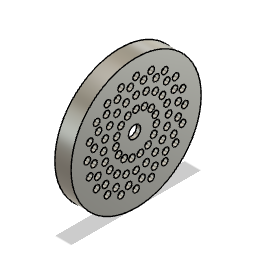
SHAPER_CAE (Autodesk Fusion 360 design; units mm, degrees)
Autodesk Fusion 360 part; units mm, degrees
sketch "Sketch1" plane through (0, 0, 0) normal (1, 0, 0) x (0, 0, -1)
  circle A0 centre (0, 0) radius 80
  circle A1 centre (0, 0) radius 70
  dimension "d1" = 160
  dimension "d2" = 140
  constraint coincident A0.centre A1.centre
  measures "d1" diameter of A0
  measures "d2" diameter of A1
extrude "Extrude1" add sketch "Sketch1" along normal blind 15
thread "Thread1" "ISO Metric profile 140.0 M140x8 6H" major diameter 140.8024 minor diameter 131.8397 pitch 8 angle 60 resizes the face on face at (10, -6.9697, -69.6522)
sketch "Sketch2" plane through (15, 0, 0) normal (1, 0, 0) x (0, 0, -1)
  circle A0 centre (0, 0) radius 65.9198
  circle A1 centre (0, 0) radius 80
  circle A2 centre (0, 0) radius 80
  constraint concentric A0 A2
extrude "Extrude2" add sketch "Sketch2" along normal blind 5 contours A0 | A1 A2
hole "Hole1" at (20, 1.6801, 1.9117) direction (-1, 0, 0) diameter 15 depth 40 tip angle 180
sketch "Sketch3" plane through (20, 0, 0) normal (1, 0, 0) x (0, 0, -1)
  circle A0 centre (-1.9117, 1.6801) radius 7.5
  circle A1 centre (0, 0) radius 80
  point P0 (0, 60)
hole "Hole2" at (20, 60, 0) direction (-1, 0, 0) diameter 8 depth 40 tip angle 180
pattern_circular "C-Pattern1" count 20 over 360 about axis through (1.75, 0, 0) along (1, 0, 0) of "Hole2"
sketch "Sketch4" plane through (20, 0, 0) normal (1, 0, 0) x (0, 0, -1)
  circle A0 centre (18.541, 57.0634) radius 4
  circle A1 centre (35.2671, 48.541) radius 4
  circle A2 centre (48.541, 35.2671) radius 4
  circle A3 centre (57.0634, 18.541) radius 4
  circle A4 centre (60, 0) radius 4
  circle A5 centre (57.0634, -18.541) radius 4
  circle A6 centre (48.541, -35.2671) radius 4
  circle A7 centre (35.2671, -48.541) radius 4
  circle A8 centre (18.541, -57.0634) radius 4
  circle A9 centre (0, -60) radius 4
  circle A10 centre (-18.541, -57.0634) radius 4
  circle A11 centre (-35.2671, -48.541) radius 4
  circle A12 centre (-48.541, -35.2671) radius 4
  circle A13 centre (-57.0634, -18.541) radius 4
  circle A14 centre (-60, 0) radius 4
  circle A15 centre (-57.0634, 18.541) radius 4
  circle A16 centre (-48.541, 35.2671) radius 4
  circle A17 centre (-35.2671, 48.541) radius 4
  circle A18 centre (-18.541, 57.0634) radius 4
  circle A19 centre (0, 60) radius 4
  circle A20 centre (-1.9117, 1.6801) radius 7.5
  circle A21 centre (0, 0) radius 80
  point P0 (-7.2239, 51.8768)
hole "Hole3" at (20, 51.8768, 7.2239) direction (-1, 0, 0) diameter 8 depth 40 tip angle 180
pattern_circular "C-Pattern2" count 20 over 360 about axis through (1.75, 0, 0) along (1, 0, 0) of "Hole3"
sketch "Sketch5" plane through (20, 0, 0) normal (1, 0, 0) x (0, 0, -1)
  circle A0 centre (9.1605, 51.5701) radius 4
  circle A1 centre (24.6482, 46.2153) radius 4
  circle A2 centre (37.7231, 36.3367) radius 4
  circle A3 centre (47.1055, 22.9012) radius 4
  circle A4 centre (51.8768, 7.2239) radius 4
  circle A5 centre (51.5701, -9.1605) radius 4
  circle A6 centre (46.2153, -24.6482) radius 4
  circle A7 centre (36.3367, -37.7231) radius 4
  circle A8 centre (22.9012, -47.1055) radius 4
  circle A9 centre (7.2239, -51.8768) radius 4
  circle A10 centre (-9.1605, -51.5701) radius 4
  circle A11 centre (-24.6482, -46.2153) radius 4
  circle A12 centre (-37.7231, -36.3367) radius 4
  circle A13 centre (-47.1055, -22.9012) radius 4
  circle A14 centre (-51.8768, -7.2239) radius 4
  circle A15 centre (-51.5701, 9.1605) radius 4
  circle A16 centre (-46.2153, 24.6482) radius 4
  circle A17 centre (-36.3367, 37.7231) radius 4
  circle A18 centre (-22.9012, 47.1055) radius 4
  circle A19 centre (-7.2239, 51.8768) radius 4
  circle A20 centre (18.541, 57.0634) radius 4
  circle A21 centre (35.2671, 48.541) radius 4
  circle A22 centre (48.541, 35.2671) radius 4
  circle A23 centre (57.0634, 18.541) radius 4
  circle A24 centre (60, 0) radius 4
  circle A25 centre (57.0634, -18.541) radius 4
  circle A26 centre (48.541, -35.2671) radius 4
  circle A27 centre (35.2671, -48.541) radius 4
  circle A28 centre (18.541, -57.0634) radius 4
  circle A29 centre (0, -60) radius 4
  circle A30 centre (-18.541, -57.0634) radius 4
  circle A31 centre (-35.2671, -48.541) radius 4
  circle A32 centre (-48.541, -35.2671) radius 4
  circle A33 centre (-57.0634, -18.541) radius 4
  circle A34 centre (-60, 0) radius 4
  circle A35 centre (-57.0634, 18.541) radius 4
  circle A36 centre (-48.541, 35.2671) radius 4
  circle A37 centre (-35.2671, 48.541) radius 4
  circle A38 centre (-18.541, 57.0634) radius 4
  circle A39 centre (0, 60) radius 4
  circle A40 centre (-1.9117, 1.6801) radius 7.5
  circle A41 centre (0, 0) radius 80
  point P0 (0, 40)
hole "Hole4" at (20, 40, 0) direction (-1, 0, 0) diameter 8 depth 40 tip angle 180
pattern_circular "C-Pattern3" count 20 over 360 about axis through (1.75, 0, 0) along (1, 0, 0) of "Hole4"
sketch "Sketch6" plane through (20, 0, 0) normal (1, 0, 0) x (0, 0, -1)
  circle A0 centre (12.3607, 38.0423) radius 4
  circle A1 centre (23.5114, 32.3607) radius 4
  circle A2 centre (32.3607, 23.5114) radius 4
  circle A3 centre (38.0423, 12.3607) radius 4
  circle A4 centre (40, 0) radius 4
  circle A5 centre (38.0423, -12.3607) radius 4
  circle A6 centre (32.3607, -23.5114) radius 4
  circle A7 centre (23.5114, -32.3607) radius 4
  circle A8 centre (12.3607, -38.0423) radius 4
  circle A9 centre (0, -40) radius 4
  circle A10 centre (-12.3607, -38.0423) radius 4
  circle A11 centre (-23.5114, -32.3607) radius 4
  circle A12 centre (-32.3607, -23.5114) radius 4
  circle A13 centre (-38.0423, -12.3607) radius 4
  circle A14 centre (-40, 0) radius 4
  circle A15 centre (-38.0423, 12.3607) radius 4
  circle A16 centre (-32.3607, 23.5114) radius 4
  circle A17 centre (-23.5114, 32.3607) radius 4
  circle A18 centre (-12.3607, 38.0423) radius 4
  circle A19 centre (0, 40) radius 4
  circle A20 centre (9.1605, 51.5701) radius 4
  circle A21 centre (24.6482, 46.2153) radius 4
  circle A22 centre (37.7231, 36.3367) radius 4
  circle A23 centre (47.1055, 22.9012) radius 4
  circle A24 centre (51.8768, 7.2239) radius 4
  circle A25 centre (51.5701, -9.1605) radius 4
  circle A26 centre (46.2153, -24.6482) radius 4
  circle A27 centre (36.3367, -37.7231) radius 4
  circle A28 centre (22.9012, -47.1055) radius 4
  circle A29 centre (7.2239, -51.8768) radius 4
  circle A30 centre (-9.1605, -51.5701) radius 4
  circle A31 centre (-24.6482, -46.2153) radius 4
  circle A32 centre (-37.7231, -36.3367) radius 4
  circle A33 centre (-47.1055, -22.9012) radius 4
  circle A34 centre (-51.8768, -7.2239) radius 4
  circle A35 centre (-51.5701, 9.1605) radius 4
  circle A36 centre (-46.2153, 24.6482) radius 4
  circle A37 centre (-36.3367, 37.7231) radius 4
  circle A38 centre (-22.9012, 47.1055) radius 4
  circle A39 centre (-7.2239, 51.8768) radius 4
  circle A40 centre (18.541, 57.0634) radius 4
  circle A41 centre (35.2671, 48.541) radius 4
  circle A42 centre (48.541, 35.2671) radius 4
  circle A43 centre (57.0634, 18.541) radius 4
  circle A44 centre (60, 0) radius 4
  circle A45 centre (57.0634, -18.541) radius 4
  circle A46 centre (48.541, -35.2671) radius 4
  circle A47 centre (35.2671, -48.541) radius 4
  circle A48 centre (18.541, -57.0634) radius 4
  circle A49 centre (0, -60) radius 4
  circle A50 centre (-18.541, -57.0634) radius 4
  circle A51 centre (-35.2671, -48.541) radius 4
  circle A52 centre (-48.541, -35.2671) radius 4
  circle A53 centre (-57.0634, -18.541) radius 4
  circle A54 centre (-60, 0) radius 4
  circle A55 centre (-57.0634, 18.541) radius 4
  circle A56 centre (-48.541, 35.2671) radius 4
  circle A57 centre (-35.2671, 48.541) radius 4
  circle A58 centre (-18.541, 57.0634) radius 4
  circle A59 centre (0, 60) radius 4
  circle A60 centre (-1.9117, 1.6801) radius 7.5
  circle A61 centre (0, 0) radius 80
  point P0 (0, 25)
hole "Hole5" at (20, 25, 0) direction (-1, 0, 0) diameter 8 depth 40 tip angle 180
pattern_circular "C-Pattern4" count 15 over 360 about axis through (1.75, 0, 0) along (1, 0, 0) of "Hole5"
mesh "Mesh1" [no effect]
